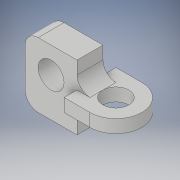
# Autodesk Inventor part: 零件22
Saved by Autodesk Inventor 2019 (Build 230136000, 136)
## iProperties
Created: 2020-09-18
Part Number: 零件22
Material: 一般
Document SubType Name: Modeling
Designer: jay
Density: 1 g/cm^3
Appearance: 預設
Author: jay
Autodesk Inventor part; units mm, degrees
ref_plane "YZ Plane" through (0, 0, 0) normal (1, 0, 0) x (0, 1, 0)
ref_plane "XZ Plane" through (0, 0, 0) normal (0, 1, 0) x (-1, 0, 0)
ref_plane "XY Plane" through (0, 0, 0) normal (0, 0, 1) x (1, 0, 0)
sketch "草圖1" plane through (0, 0, 0) normal (0, 0, 1) x (1, 0, 0)
  line L0 (0, 0) -> (40, 0)
  line L1 (40, 0) -> (40, 50)
  line L2 (40, 50) -> (0, 50)
  line L3 (0, 50) -> (0, 0)
  circle A0 centre (20, 30) radius 10
  dimension "d0" = 20
  dimension "d1" = 40
  dimension "d2" = 50
  dimension "d3" = 20
  dimension "d4" = 30
  constraints: 8 end point, 2 parallel, 1 centre point, 1 horizontal, 1 perpendicular
  measures "d0" diameter of A0
  measures "d1" distance of L1.end L2.end
  measures "d2" distance of L0.end L1.end
  measures "d3" distance from line of L3 A0.centre
  measures "d4" distance from line of A0.centre L0
extrude "擠出1" add sketch "草圖1" along normal mid plane 20
sketch "草圖2" plane through (0, 0, 0) normal (0, 0, 1) x (1, 0, 0)
  line L0 (40, 0) -> (40, 50) projected
  line L1 (40, 30) -> (80, 30)
  line L2 (80, 30) -> (80, 20)
  line L3 (80, 20) -> (40, 20)
  line L4 (40, 20) -> (40, 30)
  line L5 (0, 0) -> (40, 0) projected
  dimension "d7" = 20
  dimension "d8" = 10
  dimension "d9" = 40
  constraints: 8 end point, 2 parallel, 1 horizontal, 1 perpendicular, 1 point on line
  measures "d7" distance between parallel lines of L5 L3
  measures "d8" distance of L1.end L2.end
  measures "d9" distance of L1.start L1.end
extrude "擠出2" add sketch "草圖2" along normal mid plane 40
fillet "圓角1" radius 20 2 edges at (80, 25, -20) (80, 25, 20)
fillet "圓角2" radius 10 2 edges at (40, 30, 0) (40, 20, 0)
fillet "圓角3" radius 10 2 edges at (0, 50, 0) (0, 0, 0)
sketch "草圖3" plane through (40, 30, 20) normal (0, 1, 0) x (1, 0, 0)
  arc A0 (20, 0) -> (20, 40) centre (20, 20) ccw projected
  point P0 (-40, 20)
  constraints: 1 coincident
hole "孔1" at (60, 30, 0) direction (0, -1, 0) diameter 20 end through all
